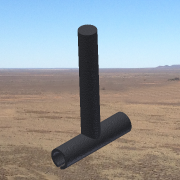
# Autodesk Inventor part: centerSpike
Saved by Autodesk Inventor 2014 SP1 (Build 180222100, 222)
## iProperties
Created: 2015-06-04
Part Number: centerSpike
Material: Iron, Cast
Document SubType Name: Modeling
Designer: Dave
Density: 7.25 g/cm^3
Appearance: Iron - Cast
Mass: 227.917 g
Surface Area: 134.524 cm^2
Volume: 31.4368 cm^3
Author: Dave
Autodesk Inventor part; units mm, degrees
ref_plane "YZ Plane" through (0, 0, 0) normal (1, 0, 0) x (0, 1, 0)
ref_plane "XZ Plane" through (0, 0, 0) normal (0, 1, 0) x (-1, 0, 0)
sketch "Sketch1" plane through (0, 0, 0) normal (0, 0, 1) x (1, 0, 0)
  circle A0 centre (0.3685, 0) radius 9.525
  circle A1 centre (0.3685, 0) radius 6.985
  point P0 (0, 0)
  dimension "d0" = 19.05
  dimension "d1" = 2.54
  constraints: 2 centre point
  measures "d0" diameter of A0
  measures "d1" radial gap between concentric circles of A1 A0
extrude "Extrusion1" add sketch "Sketch1" along normal blind 76.2
sketch "Sketch2" plane through (0.3685, 0, 76.2) normal (0, 0, 1) x (1, 0, 0)
  circle A0 centre (0, 0) radius 6.985 projected
  circle A1 centre (0, 0) radius 9.525 projected
  point P0 (-0.3685, 0)
  point P1 (-0.3685, 9.5179)
  constraints: 2 other
ref_plane "Work Plane1" through (0, 9.5179, 76.2) normal (-0.0386902, 0.9992513, 0) x (-0.9992513, -0.0386902, 0)
sketch "Sketch3" plane through (0, 9.5179, 76.2) normal (-0.0386902, 0.9992513, 0) x (-0.9992513, -0.0386902, 0)
  line L0 (0.3682, 0.0009) -> (0.3682, -76.2) construction
  circle A0 centre (0.3682, -38.0996) radius 8.255
  dimension "d4" = 16.51
  constraints: 2 end point, 1 centre point, 1 midpoint, 1 vertical
  measures "d4" diameter of A0
extrude "Extrusion2" add sketch "Sketch3" along normal blind 101.6 and the other way blind 6.35
sketch "Sketch4" plane through (0.3685, 0, 76.2) normal (0, 0, 1) x (1, 0, 0)
  line L0 (-1.5078, -6.8203) -> (-1.5078, -9.4049)
  line L1 (1.4136, -9.4195) -> (1.4136, -6.8405)
  arc A0 (-1.5078, -9.4049) -> (1.4136, -9.4195) centre (0, 0) ccw
  arc A1 (1.4136, -6.8405) -> (-1.5078, -6.8203) centre (0, 0) ccw
  constraints: 4 end point, 4 point on circle, 2 centre point, 1 coincident, 1 parallel
extrude "Extrusion3" cut sketch "Sketch4" against normal blind 101.6
body "Solid1"
